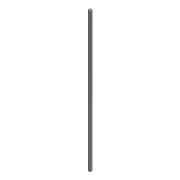
# Autodesk Inventor part: hysteresis_rod
Saved by Autodesk Inventor 2014 SP1 (Build 180222100, 222)
## iProperties
Created: 2012-08-10
Part Number: hysteresis_rod
Document SubType Name: Modeling
Designer: Robert Davis
Density: 8.74 g/cm^3
Material: Permalloy 80
Mass: 4.84381 g
Surface Area: 7.14054 cm^2
Volume: 0.554211 cm^3
Appearance: Steel
Author: Robert Davis
Autodesk Inventor part; units mm, degrees
ref_plane "YZ Plane" through (0, 0, 0) normal (1, 0, 0) x (0, 1, 0)
ref_plane "XZ Plane" through (0, 0, 0) normal (0, 1, 0) x (-1, 0, 0)
ref_plane "XY Plane" through (0, 0, 0) normal (0, 0, 1) x (1, 0, 0)
sketch "Sketch1" plane through (0, 0, 0) normal (0, 0, 1) x (1, 0, 0)
  circle A0 centre (0, 0) radius 0.7874
  dimension "d0" = 1.5748
  dimension "d0" = 1.5748
  constraints: 1 centre point
  measures "d0" diameter of A0
extrude "Extrusion1" add sketch "Sketch1" along normal mid plane 76.2
body "Solid1"
